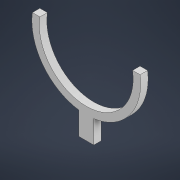
# Autodesk Inventor part: Clip_TestFitV1
Saved by Autodesk Inventor 2022 (Build 260153000, 153)
## iProperties
Created: 2023-05-05
Part Number: Clip_TestFitV1
Material: Generic
Document SubType Name: Modeling
Designer: User
Density: 1 g/cm^3
Appearance: Default
Author: User
Autodesk Inventor part; units mm, degrees
ref_plane "YZ Plane" through (0, 0, 0) normal (1, 0, 0) x (0, 1, 0)
ref_plane "XZ Plane" through (0, 0, 0) normal (0, 1, 0) x (-1, 0, 0)
ref_plane "XY Plane" through (0, 0, 0) normal (0, 0, 1) x (1, 0, 0)
sketch "Sketch1" plane through (0, 0, 0) normal (0, 0, 1) x (1, 0, 0)
  arc A0 (-31.1131, 4.9219) -> (31.1131, 4.9219) centre (0, 0) ccw
  line L0 (-31.1131, 4.9219) -> (-36.1667, 4.9219)
  line L1 (31.1131, 4.9219) -> (36.1836, 4.9349)
  line L2 (31.1131, 4.9219) -> (36.1836, 4.9349) construction
  line L3 (5.0676, -36.5047) -> (5.0676, -51.5047)
  line L4 (5.0676, -51.5047) -> (-4.9324, -51.5047)
  line L5 (-4.9324, -51.5047) -> (-4.9324, -36.5047)
  line L6 (-4.9324, -36.5047) -> (-4.9324, -36.1653)
  line L7 (5.0676, -36.5047) -> (5.0676, -36.1653)
  arc A1 (-36.1667, 4.9219) -> (-4.9324, -36.1653) centre (0, 0) ccw
  arc A2 (5.0676, -36.1653) -> (36.1836, 4.9349) centre (0, 0) ccw
  dimension "d0" = 63
  dimension "d5" = 10
  dimension "d6" = 15
  constraints: 16 end point, 6 point on circle, 3 centre point, 2 coincident, 1 parallel, 1 vertical
  measures "d0" diameter of A0
  measures "d5" distance of L3.end L4.end
  measures "d6" distance of L3.start L3.end
extrude "Extrusion1" add sketch "Sketch1" along normal blind 5
body "Solid1"
